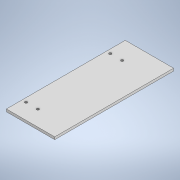
# Autodesk Inventor part: Rcr_sidewall_chasis
Saved by Autodesk Inventor 2022.2 (Build 262287000, 287)
## iProperties
Created: 2022-02-08
Part Number: Rcr_sidewall_chasis
Material: Generic
Document SubType Name: Modeling
Designer: jninj
Density: 1 g/cm^3
Appearance: Default
Author: jninj
Autodesk Inventor part; units mm, degrees
ref_plane "YZ Plane" through (0, 0, 0) normal (1, 0, 0) x (0, 1, 0)
ref_plane "XZ Plane" through (0, 0, 0) normal (0, 1, 0) x (-1, 0, 0)
ref_plane "XY Plane" through (0, 0, 0) normal (0, 0, 1) x (1, 0, 0)
sketch "Sketch1" plane through (0, 0, 0) normal (0, 1, 0) x (-1, 0, 0)
  line L0 (0, 0) -> (-123.825, 0)
  line L1 (-123.825, 0) -> (-123.825, -304.8)
  line L2 (-123.825, -304.8) -> (0, -304.8)
  line L3 (0, -304.8) -> (0, 0)
  circle A0 centre (-10.3632, -39.878) radius 3.175
  circle A1 centre (-40.6908, -39.878) radius 3.175
  circle A2 centre (-10.3632, -255.9304) radius 3.1782
  circle A3 centre (-40.6908, -255.9304) radius 3.175
  dimension "d0" = 304.8
  dimension "d1" = 123.825
  dimension "d2" = 6.35
  dimension "d3" = 6.35
  dimension "d4" = 39.878
  dimension "d5" = 39.878
  dimension "d6" = 10.3632
  dimension "d7" = 40.6908
  dimension "d8" = 10.3632
  dimension "d9" = 40.6908
  dimension "d10" = 255.9304
  dimension "d11" = 255.9304
  constraints: 8 end point, 4 centre point, 2 parallel, 1 horizontal, 1 perpendicular
  measures "d0" distance of L1.end L0.end
  measures "d1" distance of L1.end L2.end
  measures "d2" diameter of A0
  measures "d3" diameter of A1
  measures "d4" distance from line of L0 A0.centre
  measures "d5" distance from line of L0 A1.centre
  measures "d6" distance from line of L3 A0.centre
  measures "d7" distance from line of L3 A1.centre
  measures "d8" distance from line of L3 A2.centre
  measures "d9" distance from line of L3 A3.centre
  measures "d10" distance from line of L0 A3.centre
  measures "d11" distance from line of L0 A2.centre
extrude "Extrusion1" add sketch "Sketch1" along normal blind 6.35
body "Solid1"
